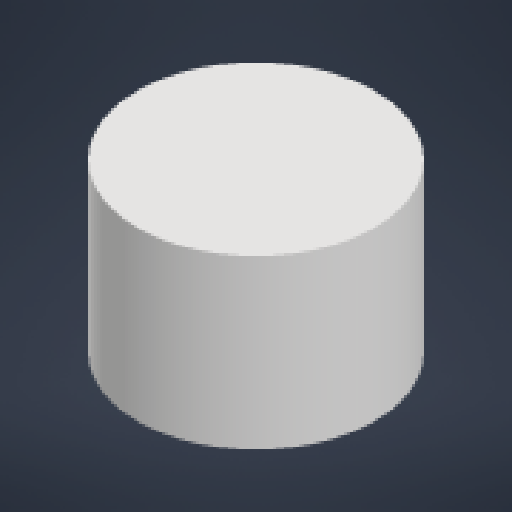
# Autodesk Inventor part: WheelBracketScrew
Saved by Autodesk Inventor 2027 (Build 310192000, 192)
## iProperties
Created: 2026-07-07
Part Number: WheelBracketScrew
Material: Generic
Document SubType Name: Modeling
Designer: belcz
Density: 1 g/cm^3
Appearance: Default
Author: belcz
Autodesk Inventor part; units mm, degrees
ref_plane "YZ Plane" through (0, 0, 0) normal (1, 0, 0) x (0, 1, 0)
ref_plane "XZ Plane" through (0, 0, 0) normal (0, 1, 0) x (-1, 0, 0)
ref_plane "XY Plane" through (0, 0, 0) normal (0, 0, 1) x (1, 0, 0)
sketch "Sketch1" plane through (0, 0, 0) normal (0, 1, 0) x (-1, 0, 0)
  circle A0 centre (0, 0) radius 4.4958
  dimension "d0" = 8.9916
  constraints: 1 centre point, 1 coincident
  measures "d0" diameter of A0
extrude "Extrusion1" add sketch "Sketch1" along normal blind 6.35
sketch "Sketch2" plane through (0, 0, 0) normal (0, -1, 0) x (1, 0, 0)
  point P0 (0, 0)
sketch "Sketch4" plane through (0, 6.35, 0) normal (0, 1, 0) x (1, 0, 0)
  circle A0 centre (0, 0) radius 4.4958 projected
  line L0 (-0.8834, 2.6038) -> (1.8133, 2.067)
  line L1 (1.8133, 2.067) -> (2.6967, -0.5368)
  line L2 (2.6967, -0.5368) -> (0.8834, -2.6038)
  line L3 (0.8834, -2.6038) -> (-1.8133, -2.067)
  line L4 (-1.8133, -2.067) -> (-2.6967, 0.5368)
  line L5 (-2.6967, 0.5368) -> (-0.8834, 2.6038)
  dimension "d4" = 4.7625
  constraints: 12 end point, 1 coincident, 13 other
  measures "d4" distance between parallel lines of L4 L1
extrude "Extrusion2" cut sketch "Sketch4" against normal blind 3.175 contours L0 L1 L2 L3 L4 L5
sketch "Sketch5" plane through (0, 0, 0) normal (0, -1, 0) x (1, 0, 0)
  circle A0 centre (0, 0) radius 4.4958 projected
  circle A1 centre (0, 0) radius 2.7305
  dimension "d7" = 5.461
  constraints: 1 centre point, 1 coincident
  measures "d7" diameter of A1
extrude "Extrusion3" add sketch "Sketch5" along normal blind 26.543 contours A1
thread "Thread1" size "1/4-20 UNC" class "2A" standard "ANSI Unified Screw Threads" full length
body "Solid1"
